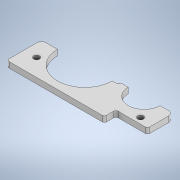
# Autodesk Inventor part: Top Bottle Front
Saved by Autodesk Inventor 2021 (Build 250183000, 183)
## iProperties
Created: 2020-09-03
Part Number: Top Bottle Front
Material: Generic
Document SubType Name: Modeling
Designer: jgray
Density: 1 g/cm^3
Appearance: Default
Author: jgray
Autodesk Inventor part; units mm, degrees
ref_plane "YZ Plane" through (0, 0, 0) normal (1, 0, 0) x (0, 1, 0)
ref_plane "XZ Plane" through (0, 0, 0) normal (0, 1, 0) x (-1, 0, 0)
ref_plane "XY Plane" through (0, 0, 0) normal (0, 0, 1) x (1, 0, 0)
sketch "Sketch1" plane through (0, 0, 0) normal (0, 1, 0) x (-1, 0, 0)
  circle A0 centre (18.5, 28) radius 23.85
  circle A1 centre (37, -23.25) radius 13.85
  circle A2 centre (-35, -38.75) radius 13.85
  circle A3 centre (-30.9, 25.8) radius 13.85
  circle A4 centre (0, -23.25) radius 13.85
  line L0 (56.25, 58.25) -> (-56.25, 58.25)
  line L1 (-56.25, -58.25) -> (56.25, -58.25)
  line L2 (0, -105.9299) -> (0, 123.2086) construction
  line L3 (-76.4777, -38.75) -> (-5.35, -38.75) construction
  line L4 (-123.5447, -23.25) -> (82.5572, -23.25) construction
  line L5 (56.25, -58.25) -> (56.25, 58.25)
  line L6 (56.25, 58.25) -> (56.25, -58.25)
  line L7 (-56.25, 58.25) -> (-56.25, -58.25)
  line L8 (100.0459, 28) -> (-13.85, 28) construction
  line L9 (-9.7154, 25.8) -> (-68.4996, 25.8) construction
  line L10 (18.5, 82.6038) -> (18.5, -4.654) construction
  line L11 (-30.9, 82.6038) -> (-30.9, 8.6393) construction
  point P0 (0, 0)
  point P1 (0, 0)
  dimension "d0" = 47.7
  dimension "d1" = 27.7
  dimension "d2" = 27.7
  dimension "d3" = 27.7
  dimension "d4" = 27.7
  dimension "d7" = 37
  dimension "d9" = 30.9
  dimension "d10" = 19.5
  dimension "d11" = 35
  dimension "d12" = 35
  dimension "d13" = 25.8
  dimension "d14" = 28
  dimension "d15" = 56.25
  dimension "d16" = 58.25
  dimension "d17" = 116.5
  dimension "d18" = 112.5
  dimension "d19" = 18.5
  dimension "d20" = 32.45
  constraints: 24 end point, 10 point on line, 5 centre point, 3 parallel, 2 horizontal, 2 perpendicular, 1 collinear, 1 vertical
  measures "d0" diameter of A0
  measures "d1" diameter of A1
  measures "d2" diameter of A2
  measures "d3" diameter of A3
  measures "d4" diameter of A4
  measures "d7" distance of A4.centre A1.centre
  measures "d9" distance from line of A3.centre L2
  measures "d10" distance between parallel lines of L1 L3
  measures "d11" distance between parallel lines of L1 L4
  measures "d12" horizontal distance of A2.centre A4.centre
  measures "d13" vertical distance of point (0, 0) A3.centre
  measures "d14" vertical distance of point (0, 0) A0.centre
  measures "d15" distance from line of point (0, 0) L5
  measures "d16" distance from line of L1 point (0, 0)
  measures "d17" distance between parallel lines of L1 L0
  measures "d18" distance between parallel lines of L7 L5
  measures "d19" horizontal distance of A0.centre point (0, 0)
  measures "d20" distance between parallel lines of L0 L9
extrude "Extrusion1" add sketch "Sketch1" along normal blind 5
sketch "Sketch2" plane through (0, 5, 0) normal (0, 1, 0) x (1, 0, 0)
  line L0 (-56.25, 58.25) -> (-56.25, -58.25) projected
  line L1 (-56.25, -58.25) -> (56.25, -58.25) projected
  line L2 (56.25, -58.25) -> (56.25, 58.25) projected
  line L3 (56.25, 58.25) -> (-56.25, 58.25) projected
  circle A0 centre (0, 23.25) radius 13.85 projected
  circle A1 centre (30.9, -25.8) radius 13.85 projected
  circle A2 centre (35, 38.75) radius 13.85 projected
  circle A3 centre (-37, 23.25) radius 13.85 projected
  circle A4 centre (-18.5, -28) radius 23.85 projected
  line L4 (-56.25, 58.25) -> (-56.25, -58.25) projected
  line L5 (-56.25, 23.25) -> (15.75, 23.25)
  line L6 (19.75, 38.75) -> (56.25, 38.75)
  line L7 (56.25, -58.25) -> (56.25, 58.25) projected
  line L8 (17.75, 25.25) -> (17.75, 36.75)
  arc A5 (15.75, 23.25) -> (17.75, 25.25) centre (15.75, 25.25) ccw
  arc A6 (19.75, 38.75) -> (17.75, 36.75) centre (19.75, 36.75) ccw
  point P0 (0, 0)
  point P1 (17.75, 23.25)
  point P2 (17.75, 38.75)
  point P3 (-50.85, 23.25)
  point P4 (-23.15, 23.25)
  point P5 (-13.85, 23.25)
  point P6 (13.85, 23.25)
  point P7 (21.15, 38.75)
  point P8 (48.85, 38.75)
  dimension "d23" = 74
  dimension "d25" = 38.5
  dimension "d26" = 2
  dimension "d27" = 35
  dimension "d28" = 19.5
  constraints: 6 end point, 6 point on line, 4 point on circle, 4 tangent, 2 centre point, 1 equal radius, 1 horizontal, 1 parallel, 1 vertical
  measures "d23" distance of point (17.75, 23.25) L5.start
  measures "d25" distance of point (17.75, 38.75) L6.end
  measures "d26" radius of A5
  measures "d27" distance between parallel lines of L3 L5
  measures "d28" distance between parallel lines of L3 L6
sketch "Sketch3" plane through (0, 5, 0) normal (0, 1, 0) x (1, 0, 0)
  line L0 (-56.25, -28) -> (8.75, -28)
  line L1 (12.3221, -25.8) -> (56.25, -25.8)
  line L2 (-56.25, 58.25) -> (-56.25, -58.25) projected
  line L3 (-56.25, -58.25) -> (56.25, -58.25) projected
  line L4 (56.25, -58.25) -> (56.25, 58.25) projected
  line L5 (56.25, 58.25) -> (-56.25, 58.25) projected
  circle A0 centre (0, 23.25) radius 13.85 projected
  circle A1 centre (30.9, -25.8) radius 13.85 projected
  circle A2 centre (35, 38.75) radius 13.85 projected
  circle A3 centre (-37, 23.25) radius 13.85 projected
  circle A4 centre (-18.5, -28) radius 23.85 projected
  line L6 (56.25, -58.25) -> (56.25, 58.25) projected
  line L7 (-56.25, 58.25) -> (-56.25, -58.25) projected
  line L8 (10.75, -26) -> (10.75, -25.8)
  arc A5 (8.75, -28) -> (10.5361, -26.9) centre (8.75, -26) ccw
  arc A6 (12.3221, -25.8) -> (10.5361, -26.9) centre (12.3221, -27.8) ccw
  point P0 (0, 0)
  point P1 (10.75, -28)
  point P2 (-42.35, -28)
  point P3 (5.35, -28)
  point P4 (17.05, -25.8)
  point P5 (44.75, -25.8)
  dimension "d29" = 67
  dimension "d30" = 2
  constraints: 7 point on line, 6 end point, 5 point on circle, 4 tangent, 2 centre point, 2 horizontal, 1 equal radius, 1 vertical
  measures "d29" distance of L0.start point (10.75, -28)
  measures "d30" radius of A5
extrude "Extrusion2" cut sketch "Sketch2" against normal through all contours L3 L2 L6 A2 A6 L8 A5 L5 A0 A3 L0
extrude "Extrusion3" cut sketch "Sketch3" against normal blind 10 contours A4 L0 L2 L5 L4 L1 A1 A6 A5
sketch "Sketch4" plane through (0, 5, 0) normal (0, 1, 0) x (1, 0, 0)
  line L0 (-56.25, -58.25) -> (56.25, -58.25) projected
  line L1 (56.25, -58.25) -> (28.75, -58.25)
  line L2 (28.75, -58.25) -> (28.75, -50.25)
  line L3 (30.75, -48.25) -> (56.25, -48.25)
  line L4 (56.25, -48.25) -> (56.25, -58.25)
  arc A0 (30.75, -48.25) -> (28.75, -50.25) centre (30.75, -50.25) ccw
  point P0 (0, 0)
  point P1 (28.75, -48.25)
  dimension "d35" = 27.5
  dimension "d36" = 10
  dimension "d37" = 2
  constraints: 8 end point, 2 parallel, 2 point on circle, 2 point on line, 2 tangent, 1 centre point, 1 horizontal, 1 perpendicular
  measures "d35" distance of point (28.75, -48.25) L3.end
  measures "d36" distance of L1.end point (28.75, -48.25)
  measures "d37" radius of A0
extrude "Extrusion4" cut sketch "Sketch4" against normal through all
sketch "Sketch5" plane through (0, 5, 0) normal (0, 1, 0) x (1, 0, 0)
  line L0 (-56.25, -28) -> (-56.25, -58.25) projected
  line L1 (56.25, -48.25) -> (56.25, -25.8) projected
  line L2 (-56.25, -58.25) -> (28.75, -58.25) projected
  line L3 (-51.25, -39.75) -> (-40.25, -39.75)
  line L4 (-40.25, -39.75) -> (-40.25, -46.75)
  line L5 (-40.25, -46.75) -> (-51.25, -46.75)
  line L6 (-51.25, -46.75) -> (-51.25, -39.75)
  line L7 (40.25, -39.75) -> (51.25, -39.75)
  line L8 (51.25, -39.75) -> (51.25, -46.75)
  line L9 (51.25, -46.75) -> (40.25, -46.75)
  line L10 (40.25, -46.75) -> (40.25, -39.75)
  point P0 (0, 0)
  point P1 (-45.25, -43.25)
  point P2 (45.25, -43.25)
  dimension "d40" = 11
  dimension "d41" = 11
  dimension "d42" = 15
  dimension "d43" = 15
  dimension "d44" = 11
  dimension "d45" = 7
  dimension "d46" = 11
  dimension "d47" = 7
  dimension "d48" = 6
  dimension "d49" = 3.5
  dimension "d50" = 6
  dimension "d51" = 3.5
  constraints: 16 end point, 4 parallel, 2 horizontal, 2 perpendicular, 1 point on line
  measures "d40" distance from line of L0 point (-45.25, -43.25)
  measures "d41" distance from line of L1 point (45.25, -43.25)
  measures "d42" distance from line of point (45.25, -43.25) L2
  measures "d43" distance from line of point (-45.25, -43.25) L2
  measures "d44" distance of L4.end L5.end
  measures "d45" distance of L3.end L4.end
  measures "d46" distance of L8.end L9.end
  measures "d47" distance of L7.end L8.end
  measures "d48" distance from line of point (-45.25, -43.25) L6
  measures "d49" distance from line of point (-45.25, -43.25) L3
  measures "d50" distance from line of L8 point (45.25, -43.25)
  measures "d51" distance from line of L7 point (45.25, -43.25)
hole "Hole1" at (-45.25, 5, 43.25) at (45.25, 5, 43.25) direction (0, -1, 0) diameter 5.1 end through all
fillet "Fillet1" radius 4 2 edges at (-56.25, 2.5, 28) (56.25, 2.5, 25.8)
fillet "Fillet2" radius 2 3 edges at (-56.25, 2.5, 58.25) (28.75, 2.5, 58.25) (56.25, 2.5, 48.25)
body "Solid1"
